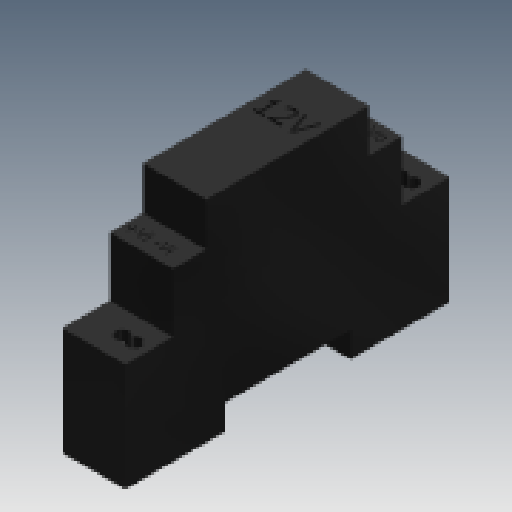
# Autodesk Inventor part: 12V_din_voltage_regulator
Saved by Autodesk Inventor 2025.4 (Build 294407020, 407B)
## iProperties
Created: 2026-09-08
Part Number: 12V_din_voltage_regulator
Material: Generic
Document SubType Name: Modeling
Designer: Aiden
Density: 1 g/cm^3
Appearance: Default
Author: Aiden
Autodesk Inventor part; units mm, degrees
ref_plane "YZ Plane" through (0, 0, 0) normal (1, 0, 0) x (0, 1, 0)
ref_plane "XZ Plane" through (0, 0, 0) normal (0, 1, 0) x (-1, 0, 0)
ref_plane "XY Plane" through (0, 0, 0) normal (0, 0, 1) x (1, 0, 0)
sketch "Sketch1" plane through (0, 0, 0) normal (0, 1, 0) x (-1, 0, 0)
  line L0 (0, 0) -> (-17.5, 0)
  line L1 (-17.5, 0) -> (-17.5, -90)
  line L2 (-17.5, -90) -> (0, -90)
  line L3 (0, -90) -> (0, 0)
  dimension "d0" = 17.5
  dimension "d1" = 90
  constraints: 8 end point, 2 parallel, 1 horizontal, 1 perpendicular
  measures "d0" distance of L1.end L2.end
  measures "d1" distance of L2.end L0.start
extrude "Extrusion1" add sketch "Sketch1" along normal blind 62.1
sketch "Sketch2" plane through (17.5, 0, 0) normal (1, 0, 0) x (0, 0, -1)
  line L0 (0, 0) -> (0, 30)
  line L1 (0, 0) -> (0, 62.1) projected
  line L2 (13.175, 30) -> (0, 30)
  line L3 (13.175, 30) -> (13.175, 46.4)
  line L4 (13.175, 46.4) -> (22.425, 46.4)
  line L5 (0, 0) -> (90, 0) projected
  line L6 (90, 0) -> (90, 62.1) projected
  line L7 (0, 62.1) -> (90, 62.1) construction
  line L8 (0, 0) -> (0, 62.1) projected
  line L9 (45, 62.1) -> (45, 0) construction
  line L10 (0, 0) -> (90, 0) projected
  line L11 (45, 0) -> (0, 0)
  line L12 (0, 62.1) -> (90, 62.1) projected
  line L13 (45, 0) -> (0, 0)
  line L14 (22.425, 46.4) -> (22.425, 58.4)
  line L15 (22.425, 58.4) -> (45, 58.4)
  line L16 (90, 0) -> (90, 62.1)
  line L17 (76.825, 30) -> (90, 30)
  line L18 (76.825, 30) -> (76.825, 46.4)
  line L19 (76.825, 46.4) -> (67.575, 46.4)
  line L20 (90, 0) -> (0, 0)
  line L21 (90, 0) -> (0, 0)
  line L22 (45, 0) -> (90, 0)
  line L23 (45, 0) -> (90, 0)
  line L24 (67.575, 46.4) -> (67.575, 58.4)
  line L25 (67.575, 58.4) -> (45, 58.4)
  point P0 (22.425, 52.4)
  point P1 (67.575, 52.4)
  point P2 (90, 30)
  dimension "d4" = 31.825
  dimension "d6" = 22.575
  dimension "d7" = 58.4
  dimension "d8" = 12
  dimension "d9" = 30
  dimension "d10" = 16.4
  constraints: 38 end point, 10 symmetric about line, 3 midpoint, 3 perpendicular, 3 point on line, 2 vertical, 1 collinear, 1 horizontal
  measures "d4" distance between parallel lines of L9 L3
  measures "d6" distance from line of L9 point (22.425, 52.4)
  measures "d7" distance between parallel lines of L11 L15
  measures "d8" distance of L4.end L14.end
  measures "d9" distance of L0.start L0.end
  measures "d10" distance of L2.start L3.end
extrude "Extrusion2" cut sketch "Sketch2" against normal through all contours L1 L12 L6 L17 L18 L19 L24 L25 L15 L14 L4 L3 L2
sketch "Sketch4" plane through (17.5, 30, -76.825) normal (0, 1, 0) x (1, 0, 0)
  line L0 (-17.5, 13.175) -> (-17.5, 0) construction
  line L1 (-17.5, 6.5875) -> (0, 6.5875) construction
  line L2 (0, -76.825) -> (0, 13.175) projected
  circle A0 centre (-7.5, 6.5875) radius 2
  circle A1 centre (-4, 6.5875) radius 2
  line L3 (-17.5, 13.175) -> (-17.5, -76.825) projected
  line L4 (-17.5, -31.825) -> (0, -31.825) construction
  circle A2 centre (-7.5, -70.2375) radius 2
  circle A3 centre (-4, -70.2375) radius 2
  point P0 (-5.75, 7.5557)
  point P1 (-5.75, 5.6193)
  point P2 (-5.75, -71.2057)
  point P3 (-5.75, -69.2693)
  dimension "d19" = 10
  dimension "d20" = 4
  dimension "d23" = 3.5
  constraints: 6 end point, 4 centre point, 3 midpoint, 2 horizontal, 2 point on line, 2 symmetric about line, 1 vertical, 4 other
  measures "d19" distance from line of L0 A0.centre
  measures "d20" diameter of A0
  measures "d23" distance of A0.centre A1.centre
extrude "Extrusion4" cut sketch "Sketch4" against normal blind 10
sketch "Sketch7" plane through (17.5, 0, 0) normal (1, 0, 0) x (0, 0, -1)
  line L0 (67.575, 58.4) -> (22.425, 58.4) projected
  line L1 (45, 58.4) -> (45, 0) construction
  line L2 (0, 0) -> (90, 0) projected
  line L3 (27.5, 7) -> (62.5, 7)
  line L4 (62.5, 7) -> (62.5, 0)
  line L5 (62.5, 0) -> (27.5, 0)
  line L6 (27.5, 0) -> (27.5, 7)
  line L7 (27.5, 7) -> (62.5, 0) construction
  line L8 (62.5, 7) -> (27.5, 0) construction
  point P0 (45, 3.5)
  dimension "d36" = 7
  dimension "d37" = 35
  constraints: 14 end point, 4 midpoint, 2 parallel, 2 point on line, 1 horizontal, 1 perpendicular
  measures "d36" distance of L5.end L3.start
  measures "d37" distance of L3.start L3.end
extrude "Extrusion5" cut sketch "Sketch7" against normal through all
sketch "Sketch5" plane through (17.5, 46.4, -67.575) normal (0, 1, 0) x (1, 0, 0)
  line L0 (-16.9536, 7.7034) -> (-0.2094, 7.7034) construction
  line L1 (-0.2094, 7.7034) -> (-0.2094, 4.5911) construction
  line L2 (-0.2094, 4.5911) -> (-16.9536, 4.5911) construction
  line L3 (-16.9536, 4.5911) -> (-16.9536, 7.7034) construction
  line L4 (-16.8858, -48.6643) -> (-0.1415, -48.6643) construction
  line L5 (-0.1415, -48.6643) -> (-0.1415, -51.7765) construction
  line L6 (-0.1415, -51.7765) -> (-16.8858, -51.7765) construction
  line L7 (-16.8858, -51.7765) -> (-16.8858, -48.6643) construction
  line L8 (-14.2243, 5.8262) -> (-15.2567, 5.8262)
  line L9 (-15.2567, 5.8262) -> (-15.2567, 4.7937)
  line L10 (-15.2567, 4.7937) -> (-15.5976, 4.7937)
  line L11 (-15.5976, 4.7937) -> (-15.5976, 5.8262)
  line L12 (-15.5976, 5.8262) -> (-16.6301, 5.8262)
  line L13 (-16.6301, 5.8262) -> (-16.6301, 6.1547)
  line L14 (-16.6301, 6.1547) -> (-15.5976, 6.1547)
  line L15 (-15.5976, 6.1547) -> (-15.5976, 7.1871)
  line L16 (-15.5976, 7.1871) -> (-15.2567, 7.1871)
  line L17 (-15.2567, 7.1871) -> (-15.2567, 6.1547)
  line L18 (-15.2567, 6.1547) -> (-14.2243, 6.1547)
  line L19 (-14.2243, 6.1547) -> (-14.2243, 5.8262)
  line L20 (-11.3838, 7.7034) -> (-12.4335, 4.6554)
  line L21 (-12.4335, 4.6554) -> (-12.8707, 4.6554)
  line L22 (-12.8707, 4.6554) -> (-13.9205, 7.7034)
  line L23 (-13.9205, 7.7034) -> (-13.4857, 7.7034)
  line L24 (-13.4857, 7.7034) -> (-12.641, 5.1716)
  line L25 (-12.641, 5.1716) -> (-11.7963, 7.7034)
  line L26 (-11.7963, 7.7034) -> (-11.3838, 7.7034)
  spline S0 degree 2 poles (-9.2423, 5.799) (-9.2423, 5.221) (-9.798, 4.5911) (-10.2624, 4.5911) knots 0 0 0 1 2 2 2
  spline S1 degree 2 poles (-10.2624, 4.5911) (-10.7391, 4.5911) (-11.285, 5.2408) (-11.285, 5.799) knots 0 0 0 1 2 2 2
  spline S2 degree 2 poles (-11.285, 5.799) (-11.285, 6.372) (-10.7218, 7.0068) (-10.2624, 7.0068) knots 0 0 0 1 2 2 2
  spline S3 degree 2 poles (-10.2624, 7.0068) (-9.798, 7.0068) (-9.2423, 6.3745) (-9.2423, 5.799) knots 0 0 0 1 2 2 2
  spline S4 degree 2 poles (-9.6399, 5.799) (-9.6399, 6.2436) (-9.9635, 6.6758) (-10.2624, 6.6758) knots 0 0 0 1 2 2 2
  spline S5 degree 2 poles (-10.2624, 6.6758) (-10.5612, 6.6758) (-10.8873, 6.2436) (-10.8873, 5.799) knots 0 0 0 1 2 2 2
  spline S6 degree 2 poles (-10.8873, 5.799) (-10.8873, 5.3667) (-10.5612, 4.9221) (-10.2624, 4.9221) knots 0 0 0 1 2 2 2
  spline S7 degree 2 poles (-10.2624, 4.9221) (-9.966, 4.9221) (-9.6399, 5.3593) (-9.6399, 5.799) knots 0 0 0 1 2 2 2
  line L27 (-6.4783, 5.8039) -> (-7.6318, 5.8039)
  line L28 (-7.6318, 5.8039) -> (-7.6318, 6.1744)
  line L29 (-7.6318, 6.1744) -> (-6.4783, 6.1744)
  line L30 (-6.4783, 6.1744) -> (-6.4783, 5.8039)
  line L31 (-3.7761, 7.7034) -> (-4.8259, 4.6554)
  line L32 (-4.8259, 4.6554) -> (-5.2631, 4.6554)
  line L33 (-5.2631, 4.6554) -> (-6.3128, 7.7034)
  line L34 (-6.3128, 7.7034) -> (-5.8781, 7.7034)
  line L35 (-5.8781, 7.7034) -> (-5.0333, 5.1716)
  line L36 (-5.0333, 5.1716) -> (-4.1886, 7.7034)
  line L37 (-4.1886, 7.7034) -> (-3.7761, 7.7034)
  spline S8 degree 2 poles (-1.6346, 5.799) (-1.6346, 5.221) (-2.1904, 4.5911) (-2.6547, 4.5911) knots 0 0 0 1 2 2 2
  spline S9 degree 2 poles (-2.6547, 4.5911) (-3.1314, 4.5911) (-3.6773, 5.2408) (-3.6773, 5.799) knots 0 0 0 1 2 2 2
  spline S10 degree 2 poles (-3.6773, 5.799) (-3.6773, 6.372) (-3.1141, 7.0068) (-2.6547, 7.0068) knots 0 0 0 1 2 2 2
  spline S11 degree 2 poles (-2.6547, 7.0068) (-2.1904, 7.0068) (-1.6346, 6.3745) (-1.6346, 5.799) knots 0 0 0 1 2 2 2
  spline S12 degree 2 poles (-2.0323, 5.799) (-2.0323, 6.2436) (-2.3559, 6.6758) (-2.6547, 6.6758) knots 0 0 0 1 2 2 2
  spline S13 degree 2 poles (-2.6547, 6.6758) (-2.9536, 6.6758) (-3.2796, 6.2436) (-3.2796, 5.799) knots 0 0 0 1 2 2 2
  spline S14 degree 2 poles (-3.2796, 5.799) (-3.2796, 5.3667) (-2.9536, 4.9221) (-2.6547, 4.9221) knots 0 0 0 1 2 2 2
  spline S15 degree 2 poles (-2.6547, 4.9221) (-2.3583, 4.9221) (-2.0323, 5.3593) (-2.0323, 5.799) knots 0 0 0 1 2 2 2
  line L38 (-14.1564, -50.5613) -> (-15.1889, -50.5613)
  line L39 (-15.1889, -50.5613) -> (-15.1889, -51.5938)
  line L40 (-15.1889, -51.5938) -> (-15.5297, -51.5938)
  line L41 (-15.5297, -51.5938) -> (-15.5297, -50.5613)
  line L42 (-15.5297, -50.5613) -> (-16.5622, -50.5613)
  line L43 (-16.5622, -50.5613) -> (-16.5622, -50.2328)
  line L44 (-16.5622, -50.2328) -> (-15.5297, -50.2328)
  line L45 (-15.5297, -50.2328) -> (-15.5297, -49.2003)
  line L46 (-15.5297, -49.2003) -> (-15.1889, -49.2003)
  line L47 (-15.1889, -49.2003) -> (-15.1889, -50.2328)
  line L48 (-15.1889, -50.2328) -> (-14.1564, -50.2328)
  line L49 (-14.1564, -50.2328) -> (-14.1564, -50.5613)
  line L50 (-11.3159, -48.6841) -> (-12.3656, -51.7321)
  line L51 (-12.3656, -51.7321) -> (-12.8028, -51.7321)
  line L52 (-12.8028, -51.7321) -> (-13.8526, -48.6841)
  line L53 (-13.8526, -48.6841) -> (-13.4179, -48.6841)
  line L54 (-13.4179, -48.6841) -> (-12.5731, -51.2158)
  line L55 (-12.5731, -51.2158) -> (-11.7284, -48.6841)
  line L56 (-11.7284, -48.6841) -> (-11.3159, -48.6841)
  line L57 (-10.6613, -51.7321) -> (-11.0467, -51.7321)
  line L58 (-11.0467, -51.7321) -> (-11.0467, -49.4448)
  line L59 (-11.0467, -49.4448) -> (-10.6613, -49.4448)
  line L60 (-10.6613, -49.4448) -> (-10.6613, -51.7321)
  line L61 (-10.6342, -49.0645) -> (-11.0714, -49.0645)
  line L62 (-11.0714, -49.0645) -> (-11.0714, -48.6643)
  line L63 (-11.0714, -48.6643) -> (-10.6342, -48.6643)
  line L64 (-10.6342, -48.6643) -> (-10.6342, -49.0645)
  line L65 (-7.727, -50.5835) -> (-8.8805, -50.5835)
  line L66 (-8.8805, -50.5835) -> (-8.8805, -50.213)
  line L67 (-8.8805, -50.213) -> (-7.727, -50.213)
  line L68 (-7.727, -50.213) -> (-7.727, -50.5835)
  line L69 (-5.0248, -48.6841) -> (-6.0745, -51.7321)
  line L70 (-6.0745, -51.7321) -> (-6.5117, -51.7321)
  line L71 (-6.5117, -51.7321) -> (-7.5615, -48.6841)
  line L72 (-7.5615, -48.6841) -> (-7.1267, -48.6841)
  line L73 (-7.1267, -48.6841) -> (-6.282, -51.2158)
  line L74 (-6.282, -51.2158) -> (-5.4372, -48.6841)
  line L75 (-5.4372, -48.6841) -> (-5.0248, -48.6841)
  line L76 (-4.3702, -51.7321) -> (-4.7555, -51.7321)
  line L77 (-4.7555, -51.7321) -> (-4.7555, -49.4448)
  line L78 (-4.7555, -49.4448) -> (-4.3702, -49.4448)
  line L79 (-4.3702, -49.4448) -> (-4.3702, -51.7321)
  line L80 (-4.343, -49.0645) -> (-4.7802, -49.0645)
  line L81 (-4.7802, -49.0645) -> (-4.7802, -48.6643)
  line L82 (-4.7802, -48.6643) -> (-4.343, -48.6643)
  line L83 (-4.343, -48.6643) -> (-4.343, -49.0645)
  point P0 (-17.5, -67.575)
  constraints: 4 other
emboss "Emboss1" sketch "Sketch5" operation cut depth 2 direction (0, -1, 0)
sketch "Sketch8" plane through (17.5, 58.4, -22.425) normal (0, 1, 0) x (1, 0, 0)
  line L0 (-16.0999, 34.1613) -> (-1.8775, 34.1613) construction
  line L1 (-1.8775, 34.1613) -> (-1.8775, 27.9368) construction
  line L2 (-1.8775, 27.9368) -> (-16.0999, 27.9368) construction
  line L3 (-16.0999, 27.9368) -> (-16.0999, 34.1613) construction
  line L4 (-12.2022, 27.9368) -> (-15.1761, 27.9368)
  line L5 (-15.1761, 27.9368) -> (-15.1761, 28.5593)
  line L6 (-15.1761, 28.5593) -> (-14.0695, 28.5593)
  line L7 (-14.0695, 28.5593) -> (-14.0695, 32.6447)
  line L8 (-14.0695, 32.6447) -> (-15.1761, 32.6447)
  line L9 (-15.1761, 32.6447) -> (-15.1761, 33.2029)
  spline S0 degree 2 poles (-15.1761, 33.2029) (-14.5487, 33.2029) (-13.9559, 33.5586) (-13.9164, 34.0526) knots 0 0 0 1 2 2 2
  line L10 (-13.9164, 34.0526) -> (-13.2841, 34.0526)
  line L11 (-13.2841, 34.0526) -> (-13.2841, 28.5593)
  line L12 (-13.2841, 28.5593) -> (-12.2022, 28.5593)
  line L13 (-12.2022, 28.5593) -> (-12.2022, 27.9368)
  line L14 (-7.3215, 27.9368) -> (-11.0808, 27.9368)
  line L15 (-11.0808, 27.9368) -> (-11.0808, 28.8013)
  spline S1 degree 2 poles (-11.0808, 28.8013) (-10.6757, 29.1817) (-9.9545, 29.8881) (-9.6087, 30.2685) knots 0 0 0 1 2 2 2
  spline S2 degree 2 poles (-9.6087, 30.2685) (-8.9122, 31.0342) (-8.4033, 31.9531) (-8.4033, 32.4421) knots 0 0 0 1 2 2 2
  spline S3 degree 2 poles (-8.4033, 32.4421) (-8.4033, 32.699) (-8.5614, 33.0843) (-8.7047, 33.2078) knots 0 0 0 1 2 2 2
  spline S4 degree 2 poles (-8.7047, 33.2078) (-8.8479, 33.3313) (-9.2234, 33.4548) (-9.4506, 33.4548) knots 0 0 0 1 2 2 2
  spline S5 degree 2 poles (-9.4506, 33.4548) (-9.668, 33.4548) (-10.1126, 33.3462) (-10.3151, 33.2622) knots 0 0 0 1 2 2 2
  spline S6 degree 2 poles (-10.3151, 33.2622) (-10.488, 33.193) (-10.8091, 32.9954) (-10.9079, 32.9263) knots 0 0 0 1 2 2 2
  line L16 (-10.9079, 32.9263) -> (-10.9524, 32.9263)
  line L17 (-10.9524, 32.9263) -> (-10.9524, 33.7957)
  spline S7 degree 2 poles (-10.9524, 33.7957) (-10.7004, 33.9192) (-9.7964, 34.1613) (-9.3913, 34.1613) knots 0 0 0 1 2 2 2
  spline S8 degree 2 poles (-9.3913, 34.1613) (-8.5367, 34.1613) (-7.5734, 33.2572) (-7.5734, 32.4866) knots 0 0 0 1 2 2 2
  spline S9 degree 2 poles (-7.5734, 32.4866) (-7.5734, 32.126) (-7.7414, 31.5233) (-7.8896, 31.2664) knots 0 0 0 1 2 2 2
  spline S10 degree 2 poles (-7.8896, 31.2664) (-8.0378, 30.9996) (-8.4676, 30.476) (-8.7047, 30.2241) knots 0 0 0 1 2 2 2
  spline S11 degree 2 poles (-8.7047, 30.2241) (-9.09, 29.8042) (-10.0335, 28.9051) (-10.3151, 28.6432) knots 0 0 0 1 2 2 2
  line L18 (-10.3151, 28.6432) -> (-7.3215, 28.6432)
  line L19 (-7.3215, 28.6432) -> (-7.3215, 27.9368)
  line L20 (-1.9121, 34.0328) -> (-4.0116, 27.9368)
  line L21 (-4.0116, 27.9368) -> (-4.886, 27.9368)
  line L22 (-4.886, 27.9368) -> (-6.9855, 34.0328)
  line L23 (-6.9855, 34.0328) -> (-6.1161, 34.0328)
  line L24 (-6.1161, 34.0328) -> (-4.4266, 28.9693)
  line L25 (-4.4266, 28.9693) -> (-2.7371, 34.0328)
  line L26 (-2.7371, 34.0328) -> (-1.9121, 34.0328)
  point P0 (-17.5, -22.425)
  constraints: 2 other
emboss "Emboss3" sketch "Sketch8" operation cut depth 2 direction (0, -1, 0)
equation "\"d30\" = d16"
equation "\"d16\" = 10"
body "Solid1"
